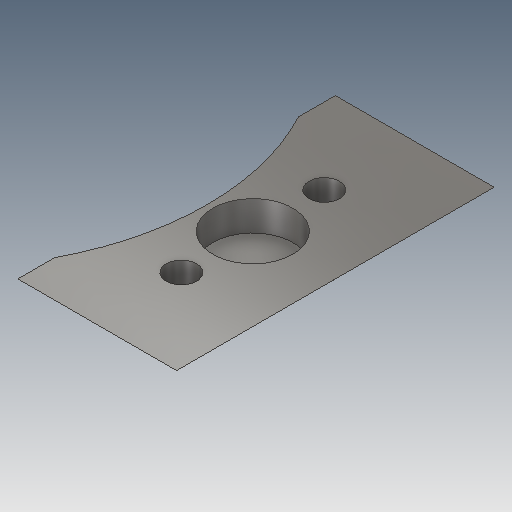
# Autodesk Inventor part: bearing_insert_thick_flat_projecting
Saved by Autodesk Inventor 2019 (Build 230136000, 136)
## iProperties
Created: 2017-07-07
Part Number: bearing_insert_thick_flat_projecting
Material: Stainless Steel, 440C
Document SubType Name: Modeling
Designer: richp
Density: 7.75 g/cm^3
Appearance: Semi-Polished
Mass: 4.40869 g
Surface Area: 7.78344 cm^2
Volume: 0.568863 cm^3
Author: richp
Autodesk Inventor part; units mm, degrees
ref_plane "YZ Plane" through (0, 0, 0) normal (1, 0, 0) x (0, 1, 0)
ref_plane "XZ Plane" through (0, 0, 0) normal (0, 1, 0) x (-1, 0, 0)
ref_plane "XY Plane" through (0, 0, 0) normal (0, 0, 1) x (1, 0, 0)
sketch "Sketch1" plane through (0, 0, 0) normal (0, 1, 0) x (-1, 0, 0)
  circle A0 centre (0, 0) radius 3.175 construction
  line L0 (3.556, 12.7) -> (-6.604, 12.7)
  line L1 (-6.604, 12.7) -> (-6.604, -12.7)
  line L2 (-6.604, -12.7) -> (3.556, -12.7)
  line L3 (3.556, -12.7) -> (3.556, 12.7)
  line L4 (5.588, 0) -> (-8.636, 0) projected
  dimension "d0" = 6.35
  dimension "d1" = 3.556
  dimension "d2" = 10.16
  dimension "d3" = 25.4
  constraints: 8 end point, 2 parallel, 1 centre point, 1 coincident, 1 horizontal, 1 perpendicular, 1 other
  measures "d0" diameter of A0
  measures "d1" distance from line of point (0, 0) L3
  measures "d2" distance between parallel lines of L1 L3
  measures "d3" distance between parallel lines of L2 L0
extrude "Extrusion1" add sketch "Sketch1" along normal blind 3.175
sketch "Sketch2" plane through (0, 3.175, 0) normal (0, 1, 0) x (1, 0, 0)
  line L0 (-5.588, 0) -> (8.636, 0) projected
  line L1 (0, 17.78) -> (0, -17.78) projected
  circle A0 centre (0, 0) radius 3.2004
  dimension "d6" = 6.4008
  constraints: 1 centre point, 1 coincident
  measures "d6" diameter of A0
extrude "Extrusion2" cut sketch "Sketch2" against normal blind 2.3813
sketch "Sketch3" plane through (0, 0, 0) normal (0, -1, 0) x (1, 0, 0)
  line L0 (0, -17.78) -> (0, 17.78) projected
  line L1 (-5.588, 0) -> (8.636, 0) projected
  point P0 (0, 0)
  point P1 (0, 5.715)
  point P2 (0, -5.715)
  dimension "d9" = 11.43
  constraints: 2 point on line, 1 symmetric about line
  measures "d9" distance of point (0, -5.715) point (0, 5.715)
hole "Hole1" at (0, 0, 5.715) at (0, 0, -5.715) direction (0, 1, 0) diameter 2.4384 depth 25.4 tip angle 118 countersink diameter 4.3688 countersink angle 82 clearance for "Flat Head Machine Screw (82)" size "#2" standard "Ansi Unified Screw Threads"
chamfer "Chamfer3" distance 3.175 angle 45 1 edges at (6.604, 0, 0)
sketch "Sketch4" plane through (0, 3.175, 0) normal (0, 1, 0) x (1, 0, 0)
  arc A0 (-3.6703, 0) -> (-7.9936, 12.7) centre (-24.4856, 0) ccw
  line L0 (-55.6819, 0) -> (16.985, 0) projected
  line L1 (-3.556, -12.7) -> (6.604, -12.7) projected
  line L2 (6.604, 12.7) -> (-3.556, 12.7) projected
  line L3 (-3.556, 12.7) -> (-3.556, -12.7) projected
  line L4 (-3.556, -12.7) -> (-7.9936, -12.7)
  line L5 (-3.556, 12.7) -> (-7.9936, 12.7)
  line L6 (-3.556, -12.7) -> (-3.556, 12.7)
  arc A1 (-7.9936, -12.7) -> (-3.6703, 0) centre (-24.4856, 0) ccw
  arc A2 (-7.9936, 12.7) -> (-7.9936, -12.7) centre (-24.4856, 0) ccw construction
  point P0 (0, 0)
  dimension "d26" = 24.4856
  dimension "d27" = 41.6306
  constraints: 6 end point, 6 point on circle, 3 centre point, 2 equal length, 2 point on line, 1 horizontal
  measures "d26" distance of point (0, 0) A0.centre
  measures "d27" diameter of A0
extrude "Extrusion3" add sketch "Sketch4" against normal blind 3.175
chamfer "Chamfer4" distance 3.175 angle 45 2 edges at (-2.282, 0, 12.7) (-2.282, 0, -12.7)
chamfer "Chamfer5" distance 0.508 angle 45 1 edges at (-3.6703, 0, 0)
sketch "Sketch5" plane through (0, 3.175, 0) normal (0, 1, 0) x (1, 0, 0)
  line L0 (-6.096, -13.97) -> (-6.096, 13.97)
  line L1 (6.604, -12.7) -> (6.604, 12.7) projected
  line L2 (-6.096, -13.97) -> (-12.446, -13.97)
  line L3 (-12.446, -13.97) -> (-12.446, 13.97)
  line L4 (-12.446, 13.97) -> (-6.096, 13.97)
  circle A0 centre (0, 0) radius 3.2004 projected
  line L5 (-16.256, 0) -> (10.414, 0) projected
  dimension "d36" = 12.7
  dimension "d37" = 6.35
  dimension "d38" = 27.94
  constraints: 8 end point, 2 perpendicular, 1 horizontal, 1 vertical, 1 other
  measures "d36" distance between parallel lines of L0 L1
  measures "d37" distance between parallel lines of L0 L3
  measures "d38" distance between parallel lines of L4 L2
extrude "Extrusion4" cut sketch "Sketch5" against normal blind 3.175 contours L2 L3 L5 L0 | L5 L3 L4 L0
sketch "Sketch6" plane through (0, 0, 0) normal (0, -1, 0) x (1, 0, 0)
  circle A0 centre (0, 0) radius 3.2004 projected
  line L0 (-5.588, 0) -> (8.636, 0) projected
  line L1 (0, -17.78) -> (0, 17.78) projected
  line L2 (0, 0) -> (2.4318, -2.8981) construction
  line L3 (-3.006, 2.3476) -> (1.79, -3.368)
  line L4 (2.3491, -3.417) -> (2.9571, -2.9067)
  line L5 (3.006, -2.3476) -> (-1.79, 3.368)
  line L6 (-2.3491, 3.417) -> (-2.9571, 2.9067)
  line L7 (-3.2612, 2.6516) -> (3.2612, -2.6516) construction
  line L8 (2.0451, -3.6721) -> (-2.0451, 3.6721) construction
  arc A1 (2.9571, -2.9067) -> (3.006, -2.3476) centre (2.702, -2.6027) ccw
  arc A2 (1.79, -3.368) -> (2.3491, -3.417) centre (2.094, -3.1129) ccw
  arc A3 (-2.9571, 2.9067) -> (-3.006, 2.3476) centre (-2.702, 2.6027) ccw
  arc A4 (-1.79, 3.368) -> (-2.3491, 3.417) centre (-2.094, 3.1129) ccw
  dimension "d41" = 50
  dimension "d42" = 8.255
  dimension "d43" = 1.5875
  dimension "d46" = 0.3969
  dimension "d47" = 140
  constraints: 14 end point, 8 point on circle, 8 point on line, 8 tangent, 4 centre point, 3 equal radius, 2 midpoint, 2 parallel, 1 perpendicular
  measures "d41" angle of L0 L2
  measures "d42" distance between parallel lines of L6 L4
  measures "d43" distance between parallel lines of L5 L3
  measures "d46" radius of A1
  measures "d47" angle of L1 L5
extrude "Extrusion5" [suppressed]
equation "\"d4\" = bearing_thickness"
equation "\"d28\" = bearing_thickness"
equation "\"d39\" = bearing_thickness"
equation "\"bearing_thickness\" = 3.175"
body "Solid1"
